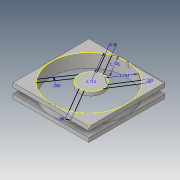
# Autodesk Inventor part: fan shell
Saved by Autodesk Inventor 2016 (Build 200138000, 138)
## iProperties
Created: 2016-05-25
Part Number: fan shell
Material: Generic
Document SubType Name: Modeling
Designer: pltwstudent
Density: 1 g/cm^3
Appearance: Default
Author: pltwstudent
Autodesk Inventor part; units mm, degrees
ref_plane "YZ Plane" through (0, 0, 0) normal (1, 0, 0) x (0, 1, 0)
ref_plane "XZ Plane" through (0, 0, 0) normal (0, 1, 0) x (-1, 0, 0)
ref_plane "XY Plane" through (0, 0, 0) normal (0, 0, 1) x (1, 0, 0)
sketch "Sketch1" plane through (0, 0, 0) normal (0, 1, 0) x (-1, 0, 0)
  line L0 (0, 0) -> (0, -139.7)
  line L1 (0, -139.7) -> (139.7, -139.7)
  line L2 (139.7, -139.7) -> (139.7, 0)
  line L3 (139.7, 0) -> (0, 0)
  dimension "d0" = 139.7
  dimension "d1" = 139.7
  dimension "d2" = 139.7
  constraints: 8 end point, 2 perpendicular, 1 vertical
  measures "d0" distance of L0.start L0.end
  measures "d1" distance of L0.end L1.end
  measures "d2" distance of L1.end L2.end
extrude "Extrusion1" add sketch "Sketch1" along normal blind 7.62
sketch "Sketch2" plane through (0, 7.62, 0) normal (0, 1, 0) x (1, 0, 0)
  line L0 (-138.43, 1.27) -> (-1.27, 1.27)
  line L1 (-1.27, 1.27) -> (-1.27, 138.43)
  line L2 (-1.27, 138.43) -> (-138.43, 138.43)
  line L3 (-138.43, 138.43) -> (-138.43, 1.27)
  line L4 (-139.7, 0) -> (0, 0) projected
  line L5 (0, 0) -> (0, 139.7) projected
  dimension "d5" = 137.16
  dimension "d6" = 137.16
  dimension "d7" = 1.27
  dimension "d8" = 1.27
  constraints: 8 end point, 2 parallel, 1 horizontal, 1 perpendicular
  measures "d5" distance of L1.end L2.end
  measures "d6" distance of L2.end L0.start
  measures "d7" distance between parallel lines of L4 L0
  measures "d8" distance between parallel lines of L1 L5
extrude "Extrusion2" cut sketch "Sketch2" against normal blind 25.4
sketch "Sketch3" plane through (0, 7.62, 0) normal (0, 1, 0) x (1, 0, 0)
  circle A0 centre (-69.85, 69.85) radius 69.85
  line L0 (-139.7, 0) -> (0, 0) projected
  line L1 (-139.7, 139.7) -> (-139.7, 0) projected
  dimension "d11" = 139.7
  dimension "d12" = 69.85
  dimension "d13" = 69.85
  constraints: 1 centre point
  measures "d11" diameter of A0
  measures "d12" distance from line of L0 A0.centre
  measures "d13" distance from line of L1 A0.centre
extrude "Extrusion3" add sketch "Sketch3" along normal blind 10.16 contours A0
sketch "Sketch4" plane through (-69.85, 17.78, -69.85) normal (0, 1, 0) x (1, 0, 0)
  line L0 (-69.85, -69.7094) -> (69.85, -69.7094)
  line L1 (69.85, -69.7094) -> (69.85, 69.9906)
  line L2 (69.85, 69.9906) -> (-69.85, 69.9906)
  line L3 (-69.85, 69.9906) -> (-69.85, -69.7094)
  line L4 (-68.58, -68.4394) -> (68.58, -68.4394)
  line L5 (68.58, -68.4394) -> (68.58, 68.7206)
  line L6 (68.58, 68.7206) -> (-68.58, 68.7206)
  line L7 (-68.58, 68.7206) -> (-68.58, -68.4394)
  point P0 (69.85, -69.85)
  dimension "d16" = 139.7
  dimension "d17" = 139.7
  dimension "d18" = 137.16
  dimension "d19" = 137.16
  dimension "d20" = 1.27
  dimension "d21" = 1.27
  constraints: 16 end point, 4 parallel, 2 horizontal, 2 perpendicular
  measures "d16" distance of L1.end L2.end
  measures "d17" distance of L0.end L1.end
  measures "d18" distance of L5.end L6.end
  measures "d19" distance of L4.end L5.end
  measures "d20" distance between parallel lines of L3 L7
  measures "d21" distance between parallel lines of L2 L6
extrude "Extrusion4" add sketch "Sketch4" along normal blind 7.62
sketch "Sketch5" plane through (0, 17.78, 0) normal (0, 1, 0) x (1, 0, 0)
  circle A0 centre (-69.85, 69.9906) radius 68.58
  line L0 (0, 0.1406) -> (0, 139.8406) projected
  line L1 (0, 139.8406) -> (-139.7, 139.8406) projected
  point P0 (0, 0)
  dimension "d24" = 137.16
  dimension "d25" = 69.85
  dimension "d26" = 69.85
  constraints: 1 centre point
  measures "d24" diameter of A0
  measures "d25" distance from line of L0 A0.centre
  measures "d26" distance from line of A0.centre L1
extrude "Extrusion5" cut sketch "Sketch5" against normal blind 25.4
sketch "Sketch6" plane through (0, 17.78, 0) normal (0, 1, 0) x (1, 0, 0)
  circle A0 centre (-69.85, 73.8341) radius 22.225
  line L0 (-139.7, 139.8406) -> (-139.7, 0.1406) projected
  point P0 (0, 0)
  dimension "d29" = 44.45
  dimension "d30" = 69.85
  constraints: 1 centre point
  measures "d29" diameter of A0
  measures "d30" distance from line of A0.centre L0
extrude "Extrusion6" add sketch "Sketch6" along normal blind 7.62
sketch "Sketch7" plane through (0, 7.62, 0) normal (0, -1, 0) x (1, 0, 0)
  line L0 (-74.2391, -138.43) -> (-138.43, -138.43) projected
  line L1 (-138.43, -138.43) -> (-138.43, -1.27) projected
  arc A0 (-138.43, -69.9906) -> (-74.2391, -138.43) centre (-69.85, -69.9906) ccw projected
  point P0 (0, 0)
extrude "Extrusion7" add sketch "Sketch7" along normal blind 7.62
sketch "Sketch8" plane through (0, 17.78, 0) normal (0, 1, 0) x (1, 0, 0)
  arc A0 (-138.43, 69.9906) -> (-1.27, 69.9906) centre (-69.85, 69.9906) ccw projected
  line L0 (-138.43, 69.9906) -> (-138.43, 1.27) projected
  line L1 (-138.43, 1.27) -> (-1.27, 1.27) projected
  arc A1 (-1.27, 69.9906) -> (-65.4609, 138.43) centre (-69.85, 69.9906) ccw projected
  line L2 (-1.27, 138.43) -> (-65.4609, 138.43) projected
  line L3 (-1.27, 1.27) -> (-1.27, 138.43) projected
  point P0 (0, 0)
extrude "Extrusion8" add sketch "Sketch8" along normal blind 7.62
sketch "Sketch9" plane through (0, 17.78, 0) normal (0, 1, 0) x (1, 0, 0)
  arc A0 (-69.85, 138.5706) -> (-138.43, 69.9906) centre (-69.85, 69.9906) ccw projected
  line L0 (-138.43, 69.9906) -> (-138.43, 138.5706) projected
  line L1 (-138.43, 138.5706) -> (-1.27, 138.5706) projected
  point P0 (0, 0)
extrude "Extrusion9" add sketch "Sketch9" along normal blind 7.62
sketch "Sketch10" plane through (0, 7.62, 0) normal (0, -1, 0) x (1, 0, 0)
  arc A0 (-1.27, -69.9906) -> (-138.43, -69.9906) centre (-69.85, -69.9906) ccw projected
  line L0 (-138.43, -1.27) -> (-1.27, -1.27) projected
  line L1 (-1.27, -1.27) -> (-1.27, -138.43) projected
  arc A1 (-138.43, -69.9906) -> (-65.4609, -138.43) centre (-69.85, -69.9906) ccw projected
  arc A2 (-65.4609, -138.43) -> (-1.27, -69.9906) centre (-69.85, -69.9906) ccw projected
  line L2 (-1.27, -138.43) -> (-65.4609, -138.43) projected
  line L3 (-138.43, -69.9906) -> (-138.43, -1.27) projected
  point P0 (0, 0)
extrude "Extrusion10" add sketch "Sketch10" along normal blind 7.62 contours A0 L3 L0 L1 | L1 L2 A2
sketch "Sketch11" plane through (-69.85, 25.4, -69.85) normal (0, 1, 0) x (1, 0, 0)
  point P0 (69.85, -69.85)
sketch "Sketch12" plane through (-69.85, 25.4, -73.8341) normal (0, 1, 0) x (1, 0, 0)
  point P0 (69.85, -73.8341)
sketch "Sketch13" plane through (-69.85, 25.4, -73.8341) normal (0, 1, 0) x (1, 0, 0)
  circle A0 centre (0, 0) radius 22.225 projected
  line L0 (-22.225, 0) -> (-53.9134, -46.2286)
  line L1 (-19.8453, -10.0057) -> (-48.9888, -52.5219)
  line L2 (22.225, 0) -> (50.003, 43.3412)
  line L3 (19.7307, 10.2298) -> (43.7736, 47.7431)
  line L4 (0, -22.225) -> (26.4575, -67.3455)
  line L5 (7.9672, -20.7479) -> (33.5583, -64.3906)
  line L6 (0, 22.225) -> (-22.6143, 60.3325)
  line L7 (-9.2826, 20.1937) -> (-31.2674, 57.6865)
  arc A1 (0, 64.7364) -> (4.3891, 64.5959) centre (0, -3.8436) ccw projected
  point P0 (69.85, -73.8341)
  dimension "d41" = 7.62
  dimension "d42" = 7.62
  dimension "d43" = 43.4631
  dimension "d44" = 44.3124
  dimension "d45" = 44.5568
  dimension "d46" = 0.3
  dimension "d47" = 7.62
  constraints: 16 end point, 3 parallel, 9 other
  measures "d41" distance between parallel lines of L5 L4
  measures "d42" distance between parallel lines of L1 L0
  measures "d43" distance of L7.start L7.end
  measures "d44" distance of L6.start L6.end
  measures "d45" distance of L3.start L3.end
  measures "d46" angle of L7 L6
  measures "d47" distance between parallel lines of L2 L3
body "Solid1"
